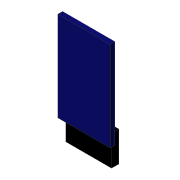
# Autodesk Inventor part: FTDI_Friend
Saved by Autodesk Inventor 2017 (Build 210142000, 142)
## iProperties
Part Number: FTDI_Friend
Material: Generisch
Document SubType Name: Modeling
Designer: Werkstatt
Density: 1 g/cm^3
Appearance: Vorgabe
Author: Werkstatt
Autodesk Inventor part; units mm, degrees
ref_plane "YZ Plane" through (0, 0, 0) normal (1, 0, 0) x (0, 1, 0)
ref_plane "XZ Plane" through (0, 0, 0) normal (0, 1, 0) x (-1, 0, 0)
ref_plane "XY Plane" through (0, 0, 0) normal (0, 0, 1) x (1, 0, 0)
sketch "Skizze1" plane through (0, 0, 0) normal (0, 1, 0) x (-1, 0, 0)
  line L0 (-8.975, 15.4) -> (8.975, 15.4)
  line L1 (8.975, 15.4) -> (8.975, -15.4)
  line L2 (8.975, -15.4) -> (-8.975, -15.4)
  line L3 (-8.975, -15.4) -> (-8.975, 15.4)
  line L4 (-8.975, 15.4) -> (8.975, -15.4) construction
  line L5 (8.975, 15.4) -> (-8.975, -15.4) construction
  point P0 (0, 0)
  dimension "d0" = 17.95
  dimension "d1" = 30.8
  constraints: 12 end point, 2 midpoint, 2 parallel, 1 horizontal, 1 perpendicular
  measures "d0" distance of L1.end L2.end
  measures "d1" distance of L0.end L1.end
extrude "Extrusion1" add sketch "Skizze1" along normal blind 1.65
sketch "Skizze2" plane through (0, 1.65, 0) normal (0, 1, 0) x (1, 0, 0)
  line L0 (-7, 5.9) -> (7, 5.9)
  line L1 (7, 5.9) -> (7, -5.9)
  line L2 (7, -5.9) -> (-7, -5.9)
  line L3 (-7, -5.9) -> (-7, 5.9)
  line L4 (-7, 5.9) -> (7, -5.9) construction
  line L5 (7, 5.9) -> (-7, -5.9) construction
  point P0 (0, 0)
  dimension "d4" = 14
  dimension "d5" = 11.8
  constraints: 12 end point, 2 midpoint, 2 parallel, 1 horizontal, 1 perpendicular
  measures "d4" distance of L1.end L2.end
  measures "d5" distance of L2.end L0.start
extrude "Extrusion2" add sketch "Skizze2" along normal blind 1.9
sketch "Skizze3" plane through (0, 1.65, 0) normal (0, 1, 0) x (1, 0, 0)
  line L0 (7, 5.9) -> (7, -5.9) projected
  line L1 (7, -5.9) -> (-7, -5.9) projected
  line L2 (-7, -5.9) -> (-7, 5.9) projected
  line L3 (-7, 5.9) -> (7, 5.9) projected
  line L4 (-8.975, -15.4) -> (8.975, -15.4) projected
  line L5 (8.975, -15.4) -> (8.975, 15.4) projected
  line L6 (8.975, 15.4) -> (-8.975, 15.4) projected
  line L7 (-8.975, 15.4) -> (-8.975, -15.4) projected
  line L8 (7.85, 12.45) -> (-7.85, 12.45)
  line L9 (-7.85, 12.45) -> (-7.85, 22.8)
  line L10 (-7.85, 22.8) -> (7.85, 22.8)
  line L11 (7.85, 22.8) -> (7.85, 12.45)
  line L12 (0, -0.0027) -> (0, 15.4) construction
  point P0 (0, 0)
  dimension "d8" = 15.7
  dimension "d9" = 2.95
  dimension "d10" = 38.2
  dimension "d11" = 10.35
  constraints: 10 end point, 2 parallel, 1 horizontal, 1 midpoint, 1 perpendicular, 1 vertical, 1 other
  measures "d8" distance of L8.start L8.end
  measures "d9" distance between parallel lines of L8 L6
  measures "d10" distance between parallel lines of L10 L4
  measures "d11" distance of L10.end L8.start
extrude "Extrusion3" add sketch "Skizze3" along normal blind 2.54 contours L9 L10 L11 L6 | L6 L11 L8 L9
